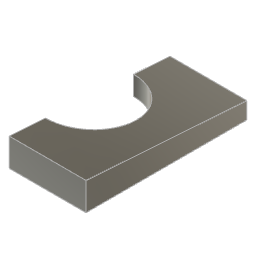
Standby Instrument Lower Support v1 (Autodesk Fusion 360 design; units mm, degrees)
Autodesk Fusion 360 part; units mm, degrees
sketch "Sketch1" plane through (0, 0, 0) normal (0, 0, 1) x (1, 0, 0)
  line L0 (0, 0) -> (11, 0)
  line L1 (11, 0) -> (11, 23)
  line L2 (11, 23) -> (0, 23)
  line L3 (0, 23) -> (0, 0)
  circle A0 centre (0, 11.5) radius 6.3012
  dimension "d1" = 11
  dimension "d2" = 23
  dimension "d3" = 12.6025
  constraint horizontal L0
  constraint vertical L1
  constraint horizontal L2
  constraint vertical L3
  constraint coincident L0.start L3.end
  constraint midpoint L3 A0.centre
  measures "d1" distance of L0.start L0.end
  measures "d2" distance of L0.start L2.end
  measures "d3" diameter of A0
extrude "Extrude1" add sketch "Sketch1" along normal blind 4 contours L0 L1 L2 L3 A0
sketch "Sketch2" plane through (11, 0, 0) normal (1, 0, 0) x (0, 1, 0)
  line L0 (0, 0) -> (23, 0)
  line L1 (23, 0) -> (23, 4)
  line L2 (23, 4) -> (0, 4)
  line L3 (0, 4) -> (0, 0)
  line L4 (0, 4) -> (23, 2.3917)
  line L5 (0, 4) -> (23.0562, 4) construction
  dimension "d6" = 4
  constraint horizontal L5
  constraint coincident L2.end L3.start
  constraint coincident L1 L4.end
  measures "d6" angle of L4 L5
extrude "Extrude2" cut sketch "Sketch2" against normal blind 14 contours L1 L2 L4
